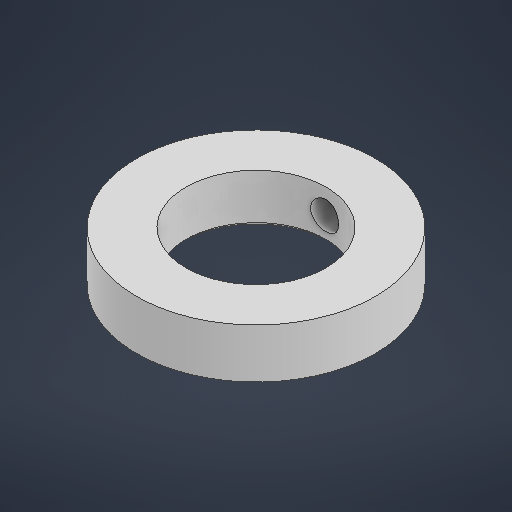
# Autodesk Inventor part: spring safety
Saved by Autodesk Inventor 2025.2 (Build 292293000, 293)
## iProperties
Created: 2025-04-19
Part Number: spring safety
Material: Generic
Document SubType Name: Modeling
Designer: klawy
Density: 1 g/cm^3
Appearance: Default
Author: klawy
Autodesk Inventor part; units mm, degrees
ref_plane "YZ Plane" through (0, 0, 0) normal (1, 0, 0) x (0, 1, 0)
ref_plane "XZ Plane" through (0, 0, 0) normal (0, 1, 0) x (-1, 0, 0)
ref_plane "XY Plane" through (0, 0, 0) normal (0, 0, 1) x (1, 0, 0)
sketch "Sketch1" plane through (0, 0, 0) normal (0, 0, 1) x (1, 0, 0)
  line L0 (8.5, 0) -> (14.5, 0)
  line L1 (14.5, 0) -> (14.5, 2.5)
  line L2 (14.5, 2.5) -> (8.5, 2.5)
  line L3 (8.5, 2.5) -> (8.5, 0)
  line L4 (8.5, 0) -> (14.5, 0)
  line L5 (14.5, 0) -> (14.5, -6)
  line L6 (14.5, -6) -> (8.5, -6)
  line L7 (8.5, -6) -> (8.5, 0)
  line L8 (0, -7.7) -> (0, 4.2) projected
  point P0 (0, 0)
  point P1 (14.5, 0)
  dimension "d0" = 2.5
  dimension "d1" = 8.5
  dimension "d2" = 6
  dimension "d3" = 6
  dimension "d4" = 6
  constraints: 16 end point, 4 parallel, 2 horizontal, 2 perpendicular, 1 point on line
  measures "d0" distance of L2.end L0.start
  measures "d1" distance from line of point (0, 0) L3
  measures "d2" distance between parallel lines of L3 L1
  measures "d3" distance of L5.end L6.end
  measures "d4" distance of L4.end L5.end
revolve "Revolution1" add sketch "Sketch1" angle 360 about axis through (0, -10, 0) along (0, 1, 0) contours L0 L5 L6 L7
sketch "Sketch2" plane through (0, 0, 0) normal (0, 0, 1) x (1, 0, 0)
  line L0 (0, 0) -> (0, -6) construction
  line L1 (8.5, -6) -> (-8.5, -6) projected
  line L2 (8.5, 0) -> (-8.5, 0) projected
  point P0 (0, -3)
  constraints: 2 end point, 2 midpoint, 1 vertical
hole "Hole1" at (0, -3, 0) direction (0, 0, -1) diameter 3.4 end through all clearance for "Hex Head Cap Screw ISO 24017" size "M3" standard "ISO"
chamfer "Chamfer1" distance 0.5 angle 45 1 edges at (-8.5, -6, 0)
body "Solid1"
